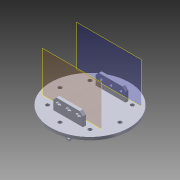
# Autodesk Inventor part: head-mount
Saved by Autodesk Inventor 2013 SP2 (Build 170200200, 200)
## iProperties
Created: 2014-11-25
Part Number: head-mount
Material: Generic
Document SubType Name: Modeling
Designer: Master
Density: 1 g/cm^3
Author: Master
Autodesk Inventor part; units mm, degrees
ref_plane "YZ Plane" through (0, 0, 0) normal (1, 0, 0) x (0, 1, 0)
ref_plane "XZ Plane" through (0, 0, 0) normal (0, 1, 0) x (-1, 0, 0)
ref_plane "XY Plane" through (0, 0, 0) normal (0, 0, 1) x (1, 0, 0)
ref_plane "Work Plane1" through (0, 0, 0) normal (0, 0, 1) x (1, 0, 0)
sketch "Sketch1" plane through (0, 0, 0) normal (0, 0, 1) x (1, 0, 0)
  line L0 (13.5, -25.5858) -> (13.5, -25) projected
  line L1 (13.5, -25.5858) -> (15, -25.5858) projected
  line L2 (15, -25.5858) -> (15, -27.5) projected
  line L3 (15.2, -27.5) -> (15, -27.5) projected
  line L4 (15.2, -27.5) -> (15.2, -27.9172) projected
  line L5 (15.2, -27.9172) -> (21.3, -27.9172) projected
  line L6 (21.3, -27.9172) -> (21.3, -25.5858) projected
  line L7 (21.3, -25.5858) -> (23.2, -25.5858) projected
  line L8 (23.2, -25.5858) -> (23.2, -27.9172) projected
  line L9 (23.2, -27.9172) -> (29.3, -27.9172) projected
  line L10 (29.3, -27.9172) -> (29.3, -25.5858) projected
  line L11 (29.3, -25.5858) -> (31.2, -25.5858) projected
  line L12 (31.2, -25.5858) -> (31.2, -27.9172) projected
  line L13 (31.2, -27.9172) -> (37.3, -27.9172) projected
  line L14 (37.3, -27.9172) -> (37.3, -25.5858) projected
  line L15 (37.3, -25.5858) -> (39.2, -25.5858) projected
  line L16 (39.2, -25.5858) -> (39.2, -27.9172) projected
  line L17 (39.2, -27.9172) -> (45.3, -27.9172) projected
  line L18 (45.3, -27.9172) -> (45.3, -26) projected
  line L19 (45.3, -26) -> (47, -26) projected
  line L20 (47, -24.5) -> (47, -26) projected
  line L21 (47, -24.5) -> (48.5, -24.5) projected
  line L22 (48.5, -24.05) -> (48.5, -24.5) projected
  line L23 (48.5, -24.05) -> (48.9172, -24.05) projected
  line L24 (48.9172, -24.05) -> (48.9172, -17.95) projected
  line L25 (48.9172, -17.95) -> (46.4172, -17.95) projected
  line L26 (46.4172, -17.95) -> (46.4172, -8.05) projected
  line L27 (46.4172, -8.05) -> (48.9172, -8.05) projected
  line L28 (48.9172, -8.05) -> (48.9172, -1.95) projected
  line L29 (48.9172, -1.95) -> (48.5, -1.95) projected
  line L30 (48.5, -1.95) -> (48.5, -1.5) projected
  line L31 (47, -1.5) -> (48.5, -1.5) projected
  line L32 (47, -1.5) -> (47, 0) projected
  line L33 (45.3, 0) -> (47, 0) projected
  line L34 (45.3, 0) -> (45.3, 1.9172) projected
  line L35 (45.3, 1.9172) -> (39.2, 1.9172) projected
  line L36 (39.2, 1.9172) -> (39.2, -0.4142) projected
  line L37 (39.2, -0.4142) -> (37.3, -0.4142) projected
  line L38 (37.3, -0.4142) -> (37.3, 1.9172) projected
  line L39 (37.3, 1.9172) -> (31.2, 1.9172) projected
  line L40 (31.2, 1.9172) -> (31.2, -0.4142) projected
  line L41 (31.2, -0.4142) -> (29.3, -0.4142) projected
  line L42 (29.3, -0.4142) -> (29.3, 1.9172) projected
  line L43 (29.3, 1.9172) -> (23.2, 1.9172) projected
  line L44 (23.2, 1.9172) -> (23.2, -0.4142) projected
  line L45 (23.2, -0.4142) -> (21.3, -0.4142) projected
  line L46 (21.3, -0.4142) -> (21.3, 1.9172) projected
  line L47 (21.3, 1.9172) -> (15.2, 1.9172) projected
  line L48 (15.2, 1.9172) -> (15.2, 1.5) projected
  line L49 (15.2, 1.5) -> (15, 1.5) projected
  line L50 (15, -0.4142) -> (15, 1.5) projected
  line L51 (15, -0.4142) -> (13.5, -0.4142) projected
  line L52 (13.5, -0.4142) -> (13.5, -1) projected
  line L53 (13.5, -1) -> (5.25, -1) projected
  line L54 (5.25, -1) -> (5.25, -3) projected
  line L55 (40.75, -3) -> (5.25, -3) projected
  arc A0 (40.7951, -3.0041) -> (40.75, -3) centre (40.75, -3.25) ccw projected
  arc A1 (43.9959, -6.2049) -> (40.7951, -3.0041) centre (43.5, -3.5) ccw projected
  arc A2 (44, -6.25) -> (43.9959, -6.2049) centre (43.75, -6.25) ccw projected
  line L56 (44, -19.75) -> (44, -6.25) projected
  arc A3 (43.9959, -19.7951) -> (44, -19.75) centre (43.75, -19.75) ccw projected
  arc A4 (40.7951, -22.9959) -> (43.9959, -19.7951) centre (43.5, -22.5) ccw projected
  arc A5 (40.75, -23) -> (40.7951, -22.9959) centre (40.75, -22.75) ccw projected
  line L57 (5.25, -23) -> (40.75, -23) projected
  line L58 (5.25, -23) -> (5.25, -25) projected
  line L59 (5.25, -25) -> (13.5, -25) projected
  line L60 (16, -27) -> (16, -26) projected
  line L61 (16, -26) -> (17.1044, -26) projected
  arc A6 (19.3956, -26) -> (17.1044, -26) centre (18.25, -26.5) ccw projected
  line L62 (19.3956, -26) -> (20.5, -26) projected
  line L63 (20.5, -26) -> (20.5, -27) projected
  line L64 (20.5, -27) -> (19.3956, -27) projected
  arc A7 (17.1044, -27) -> (19.3956, -27) centre (18.25, -26.5) ccw projected
  line L65 (17.1044, -27) -> (16, -27) projected
  line L66 (24, -27) -> (24, -26) projected
  line L67 (24, -26) -> (25.1044, -26) projected
  arc A8 (27.3956, -26) -> (25.1044, -26) centre (26.25, -26.5) ccw projected
  line L68 (27.3956, -26) -> (28.5, -26) projected
  line L69 (28.5, -26) -> (28.5, -27) projected
  line L70 (28.5, -27) -> (27.3956, -27) projected
  arc A9 (25.1044, -27) -> (27.3956, -27) centre (26.25, -26.5) ccw projected
  line L71 (25.1044, -27) -> (24, -27) projected
  line L72 (32, -27) -> (32, -26) projected
  line L73 (32, -26) -> (33.1044, -26) projected
  arc A10 (35.3956, -26) -> (33.1044, -26) centre (34.25, -26.5) ccw projected
  line L74 (35.3956, -26) -> (36.5, -26) projected
  line L75 (36.5, -26) -> (36.5, -27) projected
  line L76 (36.5, -27) -> (35.3956, -27) projected
  arc A11 (33.1044, -27) -> (35.3956, -27) centre (34.25, -26.5) ccw projected
  line L77 (33.1044, -27) -> (32, -27) projected
  line L78 (40, -27) -> (40, -26) projected
  line L79 (40, -26) -> (41.1044, -26) projected
  arc A12 (43.3956, -26) -> (41.1044, -26) centre (42.25, -26.5) ccw projected
  line L80 (43.3956, -26) -> (44.5635, -26) projected
  line L81 (44.5635, -26) -> (44.5635, -27) projected
  line L82 (44.5635, -27) -> (43.3956, -27) projected
  arc A13 (41.1044, -27) -> (43.3956, -27) centre (42.25, -26.5) ccw projected
  line L83 (41.1044, -27) -> (40, -27) projected
  line L84 (32, 1) -> (32, 0) projected
  line L85 (33.1044, 1) -> (32, 1) projected
  arc A14 (35.3956, 1) -> (33.1044, 1) centre (34.25, 0.5) ccw projected
  line L86 (36.5, 1) -> (35.3956, 1) projected
  line L87 (36.5, 0) -> (36.5, 1) projected
  line L88 (35.3956, 0) -> (36.5, 0) projected
  arc A15 (33.1044, 0) -> (35.3956, 0) centre (34.25, 0.5) ccw projected
  line L89 (32, 0) -> (33.1044, 0) projected
  line L90 (24, 1) -> (24, 0) projected
  line L91 (25.1044, 1) -> (24, 1) projected
  arc A16 (27.3956, 1) -> (25.1044, 1) centre (26.25, 0.5) ccw projected
  line L92 (28.5, 1) -> (27.3956, 1) projected
  line L93 (28.5, 0) -> (28.5, 1) projected
  line L94 (27.3956, 0) -> (28.5, 0) projected
  arc A17 (25.1044, 0) -> (27.3956, 0) centre (26.25, 0.5) ccw projected
  line L95 (24, 0) -> (25.1044, 0) projected
  line L96 (16, 1) -> (16, 0) projected
  line L97 (17.1044, 1) -> (16, 1) projected
  arc A18 (19.3956, 1) -> (17.1044, 1) centre (18.25, 0.5) ccw projected
  line L98 (20.5, 1) -> (19.3956, 1) projected
  line L99 (20.5, 0) -> (20.5, 1) projected
  line L100 (19.3956, 0) -> (20.5, 0) projected
  arc A19 (17.1044, 0) -> (19.3956, 0) centre (18.25, 0.5) ccw projected
  line L101 (16, 0) -> (17.1044, 0) projected
  line L102 (40, 1) -> (40, 0) projected
  line L103 (41.1044, 1) -> (40, 1) projected
  arc A20 (43.3956, 1) -> (41.1044, 1) centre (42.25, 0.5) ccw projected
  line L104 (44.5635, 1) -> (43.3956, 1) projected
  line L105 (44.5635, 0) -> (44.5635, 1) projected
  line L106 (43.3956, 0) -> (44.5635, 0) projected
  arc A21 (41.1044, 0) -> (43.3956, 0) centre (42.25, 0.5) ccw projected
  line L107 (40, 0) -> (41.1044, 0) projected
  line L108 (48, -7.3135) -> (48, -6.1456) projected
  line L109 (47, -7.3135) -> (48, -7.3135) projected
  line L110 (47, -6.1456) -> (47, -7.3135) projected
  arc A22 (47, -3.8544) -> (47, -6.1456) centre (47.5, -5) ccw projected
  line L111 (47, -2.6865) -> (47, -3.8544) projected
  line L112 (48, -2.6865) -> (47, -2.6865) projected
  line L113 (48, -3.8544) -> (48, -2.6865) projected
  arc A23 (48, -6.1456) -> (48, -3.8544) centre (47.5, -5) ccw projected
  line L114 (47, -18.6865) -> (48, -18.6865) projected
  line L115 (48, -18.6865) -> (48, -19.8544) projected
  arc A24 (48, -22.1456) -> (48, -19.8544) centre (47.5, -21) ccw projected
  line L116 (48, -22.1456) -> (48, -23.3135) projected
  line L117 (48, -23.3135) -> (47, -23.3135) projected
  line L118 (47, -23.3135) -> (47, -22.1456) projected
  arc A25 (47, -19.8544) -> (47, -22.1456) centre (47.5, -21) ccw projected
  line L119 (47, -19.8544) -> (47, -18.6865) projected
  circle A26 centre (18.25, -26.5) radius 1.25
  circle A27 centre (34.25, -26.5) radius 1.25
  line L120 (18.25, -26.5) -> (22.2632, -26.5) construction
  line L121 (38.25, -30) -> (38.25, -25.54)
  line L122 (35.71, -23) -> (16.79, -23)
  line L123 (14.25, -25.54) -> (14.25, -30)
  line L124 (14.25, -30) -> (38.25, -23) construction
  line L125 (38.25, -30) -> (14.25, -23) construction
  line L126 (38.25, -30) -> (38.25, -33.1242)
  line L127 (38.25, -33.1242) -> (14.25, -33.1242)
  line L128 (14.25, -33.1242) -> (14.25, -30)
  line L129 (14.25, -25.54) -> (16.79, -23)
  line L130 (35.71, -23) -> (38.25, -25.54)
  point P0 (0, 0)
  dimension "d2" = 3.1242
  constraints: 22 end point, 2 centre point, 2 coincident, 2 midpoint, 2 parallel, 1 concentric, 1 horizontal, 1 perpendicular
  measures "d2" distance of L121.start L126.end
extrude "Extrusion1" add sketch "Sketch1" along normal blind 2.3813 contours L123 L129 L57 L130 L121 L15 L14 L13 L12 L11 L10 L9 L8 L7 L6 L5 L4 L3 L2 L1 | L1 L2 L3 L4 L5 L6 L7 L8 L9 L10 L11 L12 L13 L14 L15 L121 L126 L127 L128 L123
fillet "Fillet1" radius 0.254 1 edges at (15.52, -24.27, 2.3813)
fillet "Fillet2" radius 0.254 3 edges at (26.4296, -23, 2.3813) (16.8952, -23, 2.3069) (16.79, -23, 1.0636)
fillet "Fillet3" radius 0.254 4 edges at (14.25, -27.9496, 2.3813) (14.25, -31.5621, 2.3813) (14.25, -25.6452, 2.3069) (14.25, -25.54, 1.0636)
fillet "Fillet4" radius 0.254 3 edges at (37.107, -24.397, 2.3813) (35.7844, -23.0744, 2.3069) (35.71, -23, 1.0636)
fillet "Fillet5" radius 0.254 4 edges at (38.25, -27.9496, 2.3813) (38.25, -31.5621, 2.3813) (38.25, -25.6452, 2.3069) (38.25, -25.54, 1.0636)
sketch "Sketch2" plane through (14.25, -33.1242, 0) normal (0, -1, 0) x (1, 0, 0)
  line L0 (31.75, -16.05) -> (-9.25, -16.05) projected
  line L1 (-9.25, -16.05) -> (-9.25, -26.8) projected
  line L2 (-0.75, -26.8) -> (-9.25, -26.8) projected
  line L3 (-0.75, -26.9) -> (-0.75, -26.8) projected
  line L4 (0.75, -26.9) -> (-0.75, -26.9) projected
  line L5 (0.75, -27) -> (0.75, -26.9) projected
  line L6 (0.75, -27) -> (2.8544, -27) projected
  line L7 (2.8544, -26) -> (2.8544, -27) projected
  line L8 (5.1456, -26) -> (2.8544, -26) projected
  line L9 (5.1456, -26) -> (5.1456, -27) projected
  line L10 (5.1456, -27) -> (6.25, -27) projected
  line L11 (6.25, -26.9) -> (6.25, -27) projected
  line L12 (9.75, -26.9) -> (6.25, -26.9) projected
  line L13 (9.75, -27) -> (9.75, -26.9) projected
  line L14 (9.75, -27) -> (10.8544, -27) projected
  line L15 (10.8544, -26) -> (10.8544, -27) projected
  line L16 (13.1456, -26) -> (10.8544, -26) projected
  line L17 (13.1456, -26) -> (13.1456, -27) projected
  line L18 (13.1456, -27) -> (14.25, -27) projected
  line L19 (14.25, -26.9) -> (14.25, -27) projected
  line L20 (17.75, -26.9) -> (14.25, -26.9) projected
  line L21 (17.75, -27) -> (17.75, -26.9) projected
  line L22 (17.75, -27) -> (18.8544, -27) projected
  line L23 (18.8544, -26) -> (18.8544, -27) projected
  line L24 (21.1456, -26) -> (18.8544, -26) projected
  line L25 (21.1456, -26) -> (21.1456, -27) projected
  line L26 (21.1456, -27) -> (22.25, -27) projected
  line L27 (22.25, -26.9) -> (22.25, -27) projected
  line L28 (25.75, -26.9) -> (22.25, -26.9) projected
  line L29 (25.75, -27) -> (25.75, -26.9) projected
  line L30 (25.75, -27) -> (26.8544, -27) projected
  line L31 (26.8544, -26) -> (26.8544, -27) projected
  line L32 (29.1456, -26) -> (26.8544, -26) projected
  line L33 (29.1456, -26) -> (29.1456, -27) projected
  line L34 (29.1456, -27) -> (31.75, -27) projected
  line L35 (31.75, -27) -> (31.75, -16.05) projected
  line L36 (24, 0) -> (0, 0)
  line L37 (12, 0) -> (12, -16.05)
  circle A0 centre (11.25, -16.05) radius 31.75
  line L38 (-9.25, -15.95) -> (31.75, -15.95) projected
  line L39 (31.75, -15.95) -> (31.75, -5) projected
  line L40 (29.1456, -5) -> (31.75, -5) projected
  line L41 (29.1456, -6) -> (29.1456, -5) projected
  line L42 (26.8544, -6) -> (29.1456, -6) projected
  line L43 (26.8544, -6) -> (26.8544, -5) projected
  line L44 (25.75, -5) -> (26.8544, -5) projected
  line L45 (25.75, -5) -> (25.75, -5.1) projected
  line L46 (25.75, -5.1) -> (22.25, -5.1) projected
  line L47 (22.25, -5.1) -> (22.25, -5) projected
  line L48 (21.1456, -5) -> (22.25, -5) projected
  line L49 (21.1456, -6) -> (21.1456, -5) projected
  line L50 (18.8544, -6) -> (21.1456, -6) projected
  line L51 (18.8544, -6) -> (18.8544, -5) projected
  line L52 (17.75, -5) -> (18.8544, -5) projected
  line L53 (17.75, -5) -> (17.75, -5.1) projected
  line L54 (17.75, -5.1) -> (14.25, -5.1) projected
  line L55 (14.25, -5.1) -> (14.25, -5) projected
  line L56 (13.1456, -5) -> (14.25, -5) projected
  line L57 (13.1456, -6) -> (13.1456, -5) projected
  line L58 (10.8544, -6) -> (13.1456, -6) projected
  line L59 (10.8544, -6) -> (10.8544, -5) projected
  line L60 (9.75, -5) -> (10.8544, -5) projected
  line L61 (9.75, -5) -> (9.75, -5.1) projected
  line L62 (9.75, -5.1) -> (6.25, -5.1) projected
  line L63 (6.25, -5.1) -> (6.25, -5) projected
  line L64 (5.1456, -5) -> (6.25, -5) projected
  line L65 (5.1456, -6) -> (5.1456, -5) projected
  line L66 (2.8544, -6) -> (5.1456, -6) projected
  line L67 (2.8544, -6) -> (2.8544, -5) projected
  line L68 (0.75, -5) -> (2.8544, -5) projected
  line L69 (0.75, -5) -> (0.75, -5.1) projected
  line L70 (0.75, -5.1) -> (-0.75, -5.1) projected
  line L71 (-0.75, -5.1) -> (-0.75, -5.2) projected
  line L72 (-0.75, -5.2) -> (-9.25, -5.2) projected
  line L73 (-9.25, -5.2) -> (-9.25, -15.95) projected
  point P0 (-14.25, 0)
  dimension "d14" = 63.5
  constraints: 4 end point, 2 midpoint, 2 perpendicular, 1 centre point, 1 point on line
  measures "d14" diameter of A0
extrude "Extrusion2" add sketch "Sketch2" along normal blind 2.3813 contours L35 L34 L33 L32 L31 L30 L29 L28 L27 L26 L25 L24 L23 L22 L21 L20 L19 L18 L17 L16 L15 L14 L13 L12 L11 L10 L9 L8 L7 L6 L5 L4 L3 L2 L1 L0 | L58 L57 L56 L55 L54 L53 L52 L51 L50 L49 L48 L47 L46 L45 L44 L43 L42 L41 L40 L39 L38 L37 | L37 L38 L73 L72 L71 L70 L69 L68 L67 L66 L65 L64 L63 L62 L61 L60 L59 L58 | A0
sketch "Sketch3" plane through (25.5, -35.5054, -16.05) normal (0, -1, 0) x (1, 0, 0)
  circle A0 centre (0, 0) radius 31.75 projected
  circle A1 centre (0, 24.2224) radius 1.4986
  line L0 (-10.996, 18.4312) -> (12.496, 18.4312)
  line L1 (-10.996, -18.4404) -> (12.496, -18.4404)
  line L2 (12.496, 18.4312) -> (-10.996, 18.4312)
  circle A2 centre (0, -24.2316) radius 1.4986
  line L3 (0, -24.2316) -> (0, 24.2224)
  circle A3 centre (-17.1343, -17.1343) radius 1.4986
  circle A4 centre (-24.2316, 0) radius 1.4986
  circle A5 centre (-17.1343, 17.1343) radius 1.4986
  circle A6 centre (17.1343, 17.1343) radius 1.4986
  circle A7 centre (24.2316, 0) radius 1.4986
  circle A8 centre (17.1343, -17.1343) radius 1.4986
  point P0 (-25.5, 16.05)
  dimension "d18" = 2.9972
  dimension "d21" = 2.9972
  dimension "d22" = 2.9972
  dimension "d23" = 2.9972
  dimension "d24" = 2.9972
  dimension "d25" = 2.9972
  dimension "d26" = 2.9972
  dimension "d27" = 2.9972
  constraints: 8 centre point, 8 end point, 1 coincident, 1 horizontal, 1 parallel, 1 perpendicular
  measures "d18" diameter of A1
  measures "d21" diameter of A2
  measures "d22" diameter of A3
  measures "d23" diameter of A4
  measures "d24" diameter of A5
  measures "d25" diameter of A6
  measures "d26" diameter of A7
  measures "d27" diameter of A8
extrude "Extrusion3" cut sketch "Sketch3" against normal blind 101.6 contours A1 | A2 | A3 | A4 | A5 | A6 | A7 | A8
ref_plane "Work Plane2" through (0, 0, -32) normal (0, 0, -1) x (-1, 0, 0)
sketch "Sketch4" plane through (0, 0, -32) normal (0, 0, -1) x (-1, 0, 0)
  line L0 (-17.1044, -26) -> (-16, -26) projected
  line L1 (-16, -26) -> (-16, -27) projected
  line L2 (-16, -27) -> (-17.1044, -27) projected
  arc A0 (-19.3956, -27) -> (-17.1044, -27) centre (-18.25, -26.5) ccw projected
  line L3 (-19.3956, -27) -> (-20.5, -27) projected
  line L4 (-20.5, -27) -> (-20.5, -26) projected
  line L5 (-20.5, -26) -> (-19.3956, -26) projected
  arc A1 (-17.1044, -26) -> (-19.3956, -26) centre (-18.25, -26.5) ccw projected
  line L6 (-25.1044, -26) -> (-24, -26) projected
  line L7 (-24, -26) -> (-24, -27) projected
  line L8 (-24, -27) -> (-25.1044, -27) projected
  arc A2 (-27.3956, -27) -> (-25.1044, -27) centre (-26.25, -26.5) ccw projected
  line L9 (-27.3956, -27) -> (-28.5, -27) projected
  line L10 (-28.5, -27) -> (-28.5, -26) projected
  line L11 (-28.5, -26) -> (-27.3956, -26) projected
  arc A3 (-25.1044, -26) -> (-27.3956, -26) centre (-26.25, -26.5) ccw projected
  line L12 (-33.1044, -26) -> (-32, -26) projected
  line L13 (-32, -26) -> (-32, -27) projected
  line L14 (-32, -27) -> (-33.1044, -27) projected
  arc A4 (-35.3956, -27) -> (-33.1044, -27) centre (-34.25, -26.5) ccw projected
  line L15 (-35.3956, -27) -> (-36.5, -27) projected
  line L16 (-36.5, -27) -> (-36.5, -26) projected
  line L17 (-36.5, -26) -> (-35.3956, -26) projected
  arc A5 (-33.1044, -26) -> (-35.3956, -26) centre (-34.25, -26.5) ccw projected
  arc A6 (-38.1756, -25.4656) -> (-38.25, -25.6452) centre (-37.996, -25.6452) ccw projected
  line L18 (-38.25, -25.6452) -> (-38.25, -33.1242) projected
  line L19 (-38.25, -33.1242) -> (-14.25, -33.1242) projected
  line L20 (-14.25, -33.1242) -> (-14.25, -25.6452) projected
  arc A7 (-14.25, -25.6452) -> (-14.3244, -25.4656) centre (-14.504, -25.6452) ccw projected
  line L21 (-14.3244, -25.4656) -> (-16.7156, -23.0744) projected
  arc A8 (-16.7156, -23.0744) -> (-16.8952, -23) centre (-16.8952, -23.254) ccw projected
  line L22 (-16.8952, -23) -> (-35.6048, -23) projected
  arc A9 (-35.6048, -23) -> (-35.7844, -23.0744) centre (-35.6048, -23.254) ccw projected
  line L23 (-35.7844, -23.0744) -> (-38.1756, -25.4656) projected
  circle A10 centre (-34.25, -26.5) radius 1.25
  circle A11 centre (-26.25, -26.5) radius 1.25
  circle A12 centre (-18.25, -26.5) radius 1.25
  point P0 (0, 0)
  constraints: 3 coincident, 9 other
extrude "Extrusion4" add sketch "Sketch4" along normal blind 2.3813 contours L0 L1 L2 A12 | A12 L3 L4 L5 | L6 L7 L8 A11 | A11 L9 L10 L11 | L12 L13 L14 A10 | A10 L15 L16 L17 | L23 A9 L22 A8 L21 A7 L20 L19 L18 A6
fillet "Fillet6" radius 0.254 9 edges at (35.702, -23.0193, -34.3812) (36.98, -24.27, -34.3812) (38.2307, -25.548, -34.3812) (38.25, -29.3847, -34.3812) (16.798, -23.0193, -34.3812) (15.52, -24.27, -34.3812) (14.2693, -25.548, -34.3812) (14.25, -29.3847, -34.3812) (26.25, -23, -34.3812)
sketch "Sketch5" plane through (0, 0, 2.3813) normal (0, 0, 1) x (1, 0, 0)
  line L0 (16.8952, -23.254) -> (35.6048, -23.254) projected
  line L1 (14.504, -33.1242) -> (37.996, -33.1242)
  line L2 (-6.25, -35.5054) -> (57.25, -35.5054) projected
  line L3 (57.25, -33.1242) -> (-6.25, -33.1242) projected
  circle A0 centre (26.25, -45.8242) radius 1.4986
  arc A1 (23.7423, -47.272) -> (28.7577, -47.272) centre (26.25, -45.8242) ccw
  line L4 (28.7577, -47.272) -> (37.996, -35.5054)
  line L5 (23.7423, -47.272) -> (14.504, -35.5054)
  dimension "d34" = 2.9972
  dimension "d35" = 5.7912
  constraints: 6 end point, 2 centre point, 2 point on circle, 2 point on line, 1 coincident, 1 parallel
  measures "d34" diameter of A0
  measures "d35" diameter of A1
extrude "Extrusion5" add sketch "Sketch5" against normal blind 2.3813
sketch "Sketch6" plane through (0, 0, -34.3812) normal (0, 0, -1) x (-1, 0, 0)
  circle A0 centre (-26.25, -45.8242) radius 1.4986 projected
  arc A1 (-28.7577, -47.272) -> (-23.7423, -47.272) centre (-26.25, -45.8242) ccw projected
  line L0 (-23.7423, -47.272) -> (-14.504, -35.5054) projected
  line L1 (-37.996, -35.5054) -> (-14.504, -35.5054) projected
  line L2 (-37.996, -35.5054) -> (-28.7577, -47.272) projected
  point P0 (0, 0)
extrude "Extrusion6" add sketch "Sketch6" against normal blind 2.3813
body "Solid1"
